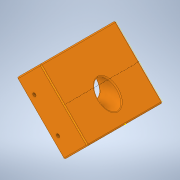
# Autodesk Inventor part: drillGuide
Saved by Autodesk Inventor 2020.1 (Build 241239000, 239)
## iProperties
Created: 2019-06-16
Part Number: drillGuide
Material: Nylon 6/6
Document SubType Name: Modeling
Designer: steele
Density: 1.13 g/cm^3
Appearance: Orange
Author: steele
Autodesk Inventor part; units mm, degrees
ref_plane "YZ Plane" through (0, 0, 0) normal (1, 0, 0) x (0, 1, 0)
ref_plane "XY Plane" through (0, 0, 0) normal (0, 0, 1) x (1, 0, 0)
sketch "Sketch1" plane through (0, 0, 0) normal (0, 0, 1) x (1, 0, 0)
  line L0 (0, 0) -> (-71.842049, 71.842049)
  line L1 (0, 0) -> (101.6, 0) construction
  line L2 (-71.842049, 71.842049) -> (-53.881537, 89.802561)
  line L3 (-71.842049, 71.842049) -> (-46.442049, 71.842049) construction
  line L4 (0, 0) -> (17.960512, 17.960512)
  line L5 (0, 0) -> (25.4, 0) construction
  line L6 (17.960512, 17.960512) -> (-53.881537, 89.802561)
  dimension "guideLength" = 101.6
  dimension "d1" = 135
  dimension "guideDepth" = 25.4
  dimension "d3" = 45
  dimension "d4" = 25.4
  dimension "d5" = 45
  constraints: 14 end point, 3 equal length, 3 horizontal, 1 perpendicular
  measures "guideLength" distance of L0.start L0.end
  measures "d1" angle of L1 L0
  measures "guideDepth" distance of L0.end L2.end
  measures "d3" angle of L3 L2
  measures "d4" distance of L0.start L4.end
  measures "d5" angle of L5 L4
extrude "Extrusion1" add sketch "Sketch1" along normal mid plane 114.3
sketch "Sketch3" plane through (-53.881537, 89.802561, -57.15) normal (0.7071068, 0.7071068, 0) x (-0.7071068, 0.7071068, 0)
  line L0 (0, 114.3) -> (-101.6, 114.3) construction
  line L1 (-50.8, 114.3) -> (-50.8, 0) construction
  line L2 (0, 0) -> (-101.6, 0) construction
  point P0 (-101.6, 57.15)
  constraints: 2 end point, 2 midpoint
ref_plane "Work Plane1" through (-17.960512, 53.881537, 57.15) normal (1, 0, 0) x (0, 0, -1)
sketch "Sketch4" plane through (-17.960512, 53.881537, 57.15) normal (1, 0, 0) x (0, 0, -1)
  line L0 (0, -35.921024) -> (0, 35.921024)
  circle A0 centre (57.15, -10.521024) radius 13.97
  line L1 (0, -35.921024) -> (114.3, -35.921024)
  point P0 (57.15, -53.881537)
  dimension "holeDiameter" = 27.94
  dimension "holeCenter" = 57.15
  dimension "d21" = 25.4
  constraints: 1 centre point
  measures "holeDiameter" diameter of A0
  measures "holeCenter" distance from line of A0.centre L0
  measures "d21" distance from line of L1 A0.centre
extrude "Extrusion2" cut sketch "Sketch4" along normal through all both and the other way through all
sketch "Sketch5" plane through (0, 0, 57.15) normal (-0.7071068, -0.7071068, 0) x (-0.7071068, 0.7071068, 0)
  line L0 (101.6, 0) -> (101.6, 114.3) construction
  line L1 (101.6, 57.15) -> (0, 57.15) construction
  line L2 (0, 114.3) -> (0, 0) projected
  line L3 (101.6, 114.3) -> (0, 114.3)
  line L4 (0, 114.3) -> (0, 101.6)
  line L5 (0, 101.6) -> (101.6, 101.6)
  line L6 (101.6, 101.6) -> (101.6, 114.3)
  line L7 (101.6, 114.3) -> (101.6, 0) construction
  line L8 (0, 0) -> (0, 114.3)
  line L9 (101.6, 0) -> (0, 0)
  line L10 (0, 12.7) -> (101.6, 12.7)
  line L11 (101.6, 12.7) -> (101.6, 0)
  dimension "guideSideRectangle" = 12.7
  constraints: 20 end point, 7 symmetric about line, 2 horizontal, 2 parallel, 2 point on line, 1 midpoint, 1 perpendicular
  measures "guideSideRectangle" distance between parallel lines of L5 L3
extrude "Extrusion3" add sketch "Sketch5" along normal blind 25.4
sketch "Sketch6" plane through (0, 0, 57.15) normal (0, 0, 1) x (1, 0, 0)
  line L0 (-71.842049, 71.842049) -> (-89.802561, 53.881537) construction
  line L1 (-80.822305, 62.861793) -> (-8.980256, -8.980256) construction
  line L2 (17.960512, 17.960512) -> (-17.960512, -17.960512) construction
  line L3 (-17.960512, -17.960512) -> (-89.802561, 53.881537)
  point P0 (0, 0)
  point P1 (-62.861793, 44.901281)
  point P2 (-26.940768, 8.980256)
  dimension "centerLineForScrews" = 12.7
  dimension "d26" = 25.4
  dimension "d27" = 25.4
  constraints: 3 point on line, 2 end point, 1 midpoint
  measures "centerLineForScrews" distance between parallel lines of L3 L1
  measures "d26" distance of L1.start point (-62.862, 44.901)
  measures "d27" distance of L1.end point (-26.941, 8.98)
hole "Hole2" at (-62.861793, 44.901281, 57.15) at (-26.940768, 8.980256, 57.15) direction (0, 0, -1) diameter 5.1054 end through all clearance for "Flat Head Machine Screw (82)" size "#10" standard "Ansi Unified Screw Threads"
fillet "Fillet1" radius 1.5875 8 edges at (-53.8815, 17.9605, 57.15) (-17.9605, -17.9605, 50.8) (-53.8815, 17.9605, 44.45) (-89.8026, 53.8815, 50.8) (-89.8026, 53.8815, -50.8) (-53.8815, 17.9605, -44.45) (-53.8815, 17.9605, -57.15) (-17.9605, -17.9605, -50.8)
fillet "Fillet2" radius 1.5875 4 edges at (0, 0, 0) (-35.921, 35.921, -44.45) (-71.842, 71.842, 0) (-35.921, 35.921, 44.45)
fillet "Fillet3" radius 1.5875 5 edges at (17.9605, 17.9605, 0) (-17.9605, -17.3029, 56.685) (0.5613, 0.5613, 57.15) (-17.9605, -17.3029, -56.685) (0.5613, 0.5613, -57.15)
fillet "Fillet4" radius 1.5875 5 edges at (-89.145, 53.8815, -56.685) (-71.2808, 72.4033, -57.15) (-53.8815, 89.8026, 0) (-89.145, 53.8815, 56.685) (-71.2808, 72.4033, 57.15)
fillet "Fillet5" radius 1.5875 6 edges at (17.3029, 17.9605, -56.685) (-53.8815, 89.145, -56.685) (-17.9605, 53.8815, -57.15) (-53.8815, 89.145, 56.685) (17.3029, 17.9605, 56.685) (-17.9605, 53.8815, 57.15)
fillet "Fillet6" radius 1.5875 4 edges at (5.2797, 30.6413, 5.7778) (-21.4095, 57.3305, 0) (-13.2173, 49.1384, -12.7192) (-43.3605, 43.3605, 13.97)
equation "\"d4\" = guideDepth"
equation "\"guideWidth\" = boardWidth + 2 * guideSideWidth"
equation "\"holeCenter\" = 0.5 * guideWidth"
equation "\"guideSideRectangle\" = guideSideWidth"
equation "\"centerLineForScrews\" = 0.5 * guideSideDepth"
equation "\"boardWidth\" = 88.9"
equation "\"guideSideWidth\" = 12.7"
equation "\"guideSideDepth\" = 25.4"
body "Solid1"
